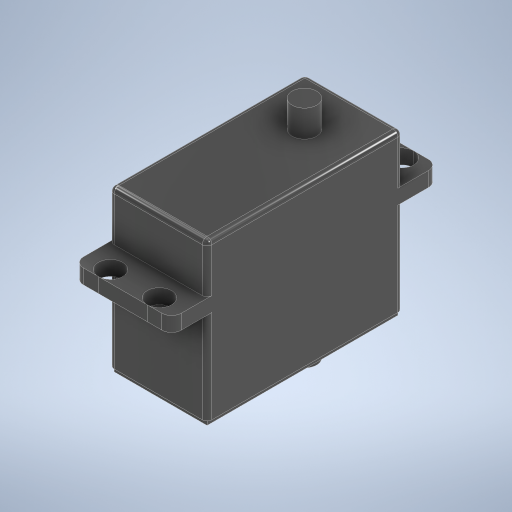
# Autodesk Inventor part: Servo40KgRough
Saved by Autodesk Inventor 2024 (Build 280153000, 153)
## iProperties
Created: 2025-12-19
Part Number: Servo40KgRough
Material: Generic
Document SubType Name: Modeling
Designer: Liam
Density: 1 g/cm^3
Appearance: Dark Gray
Author: Liam
Autodesk Inventor part; units mm, degrees
ref_plane "YZ Plane" through (0, 0, 0) normal (1, 0, 0) x (0, 1, 0)
ref_plane "XZ Plane" through (0, 0, 0) normal (0, 1, 0) x (-1, 0, 0)
ref_plane "XY Plane" through (0, 0, 0) normal (0, 0, 1) x (1, 0, 0)
sketch "Sketch1" plane through (0, 0, 0) normal (1, 0, 0) x (0, 1, 0)
  line L0 (0, 0) -> (40.5, 0)
  line L1 (40.5, 0) -> (40.5, -40)
  line L2 (40.5, -40) -> (0, -40)
  line L3 (0, -40) -> (0, 0)
  line L4 (46, -27.4) -> (40.5, -27.4)
  line L5 (40.5, -27.4) -> (40.5, -32.4)
  line L6 (40.5, -32.4) -> (46, -32.4)
  line L7 (46, -32.4) -> (46, -27.4)
  line L8 (46, -27.4) -> (40.5, -32.4) construction
  line L9 (40.5, -27.4) -> (46, -32.4) construction
  line L10 (40.5, -20) -> (0, -20) construction
  line L11 (27.5, 0) -> (30.5, 0)
  line L12 (30.5, 0) -> (30.5, 7.25)
  line L13 (30.5, 7.25) -> (27.5, 7.25)
  line L14 (27.5, 7.25) -> (27.5, 0)
  line L15 (27.5, -40) -> (30.5, -40)
  line L16 (30.5, -40) -> (30.5, -47.25)
  line L17 (30.5, -47.25) -> (27.5, -47.25)
  line L18 (27.5, -47.25) -> (27.5, -40)
  line L19 (3, -40) -> (6.5, -40)
  line L20 (6.5, -40) -> (6.5, -45.5)
  line L21 (6.5, -45.5) -> (3, -45.5)
  line L22 (3, -45.5) -> (3, -40)
  line L23 (0, -40) -> (7.5, -40)
  line L24 (7.5, -40) -> (7.5, 0)
  line L25 (7.5, 0) -> (0, 0)
  line L26 (0, 0) -> (0, -40)
  point P0 (43.25, -29.9)
  point P1 (30.5, 0)
  dimension "d0" = 40
  dimension "d1" = 40.5
  dimension "d2" = 10.1
  dimension "d3" = 5.5
  dimension "d4" = 5
  dimension "d5" = 20
  dimension "d6" = 3
  dimension "d7" = 27.5
  dimension "d8" = 7.25
  dimension "d31" = 3.5
  dimension "d32" = 5.5
  dimension "d33" = 21
  dimension "d34" = 3
  dimension "d41" = 3
  dimension "d42" = 20
  dimension "d43" = 7.5
  constraints: 54 end point, 10 parallel, 5 horizontal, 5 perpendicular, 4 midpoint, 4 point on line, 4 symmetric about line
  measures "d0" distance of L2.end L0.start
  measures "d1" distance of L1.end L2.end
  measures "d2" distance from line of L2 point (43.25, -29.9)
  measures "d3" distance of L5.end L6.end
  measures "d4" distance of L6.end L4.start
  measures "d5" distance between parallel lines of L0 L10
  measures "d6" distance of L12.end L13.end
  measures "d7" distance between parallel lines of L3 L14
  measures "d8" distance of L11.end L12.end
  measures "d31" distance of L20.end L21.end
  measures "d32" distance of L21.end L19.start
  measures "d33" distance between parallel lines of L18 L20
  measures "d34" distance between parallel lines of L22 L3
  measures "d41" distance between parallel lines of L14 L16
  measures "d42" distance between parallel lines of L18 L24
  measures "d43" distance between parallel lines of L3 L24
sketch "Sketch2" plane through (0, 0, 0) normal (0, 1, 0) x (-1, 0, 0)
  line L0 (0, 0) -> (20, 0)
  line L1 (20, 0) -> (20, -40)
  line L2 (20, -40) -> (0, -40)
  line L3 (0, -40) -> (0, 0)
  line L4 (0, 0) -> (20, 0)
  line L5 (20, 0) -> (20, 7.25)
  line L6 (20, 7.25) -> (0, 7.25)
  line L7 (0, 7.25) -> (0, 0)
  circle A0 centre (5, 4.75) radius 2.5
  line L8 (10, 7.25) -> (10, 0) construction
  circle A1 centre (15, 4.75) radius 2.5
  line L9 (20, -20) -> (0, -20) construction
  line L10 (20, -40) -> (20, -47.25)
  line L11 (20, -47.25) -> (0, -47.25)
  line L12 (0, -47.25) -> (0, -40)
  circle A2 centre (5, -44.75) radius 2.5
  circle A3 centre (15, -44.75) radius 2.5
  circle A4 centre (10, -29.9) radius 2.5
  line L13 (0, -0.5) -> (19.5, -0.5)
  line L14 (19.5, -0.5) -> (19.5, -39.5)
  line L15 (19.5, -39.5) -> (0, -39.5)
  line L16 (0.5, -40) -> (0.5, 0)
  point P0 (0.5, -0.5)
  point P1 (0.5, -39.5)
  dimension "d9" = 40
  dimension "d10" = 20
  dimension "d11" = 7.25
  dimension "d12" = 20
  dimension "d13" = 5
  dimension "d14" = 5
  dimension "d15" = 2.5
  dimension "d16" = 5
  dimension "d17" = 10.1
  dimension "d18" = 10
  dimension "d19" = 14.85
  dimension "d20" = 34.65
  dimension "d21" = 54.5
  dimension "d30" = 49.5
  dimension "d44" = 0.5
  dimension "d45" = 0.5
  constraints: 34 end point, 6 parallel, 6 symmetric about line, 5 centre point, 4 midpoint, 3 perpendicular, 2 horizontal, 5 other
  measures "d9" distance of L2.end L0.start
  measures "d10" distance of L1.end L2.end
  measures "d11" distance of L4.end L5.end
  measures "d12" distance of L5.end L6.end
  measures "d13" diameter of A0
  measures "d14" distance from line of L8 A0.centre
  measures "d15" distance from line of L6 A0.centre
  measures "d16" diameter of A4
  measures "d17" distance from line of L2 A4.centre
  measures "d18" distance from line of L3 A4.centre
  measures "d19" vertical distance of A4.centre A3.centre
  measures "d20" vertical distance of A1.centre A4.centre
  measures "d21" distance between parallel lines of L11 L6
  measures "d30" distance of A0.centre A2.centre
  measures "d44" distance between parallel lines of L3 L16
  measures "d45" distance between parallel lines of L0 L13
extrude "Extrusion1" add sketch "Sketch1" against normal blind 20 contours L0 L1 L2 L24 | L14 L13 L12 L0 | L2 L16 L17 L18
extrude "Extrusion2" cut sketch "Sketch2" along normal blind 100 contours A1 | A0 | A2 | A3
extrude "Extrusion3" add sketch "Sketch2" along normal blind 46 contours A4
fillet "Fillet1" radius 2 4 edges at (-20, 29, 7.25) (0, 29, 7.25) (0, 29, -47.25) (-20, 29, -47.25)
fillet "Fillet2" radius 1 12 edges at (0, 17.5, 0) (0, 35.5, 0) (0, 35.5, -40) (0, 17.5, -40) (-20, 35.5, -40) (-20, 17.5, -40) (-20, 35.5, 0) (-20, 17.5, 0) (-20, 40.5, -20) (-10, 40.5, 0) (0, 40.5, -20) (-10, 40.5, -40)
extrude "Extrusion5" cut sketch "Sketch2" along normal blind 8.5 contours L0 L16 L13 L3 | L0 L1 L2 L16 L15 L14 L13 | L13 L16 L15 L3 | L15 L16 L2 L3
body "Solid1"
